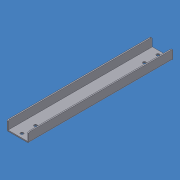
# Autodesk Inventor part: schuivend U-profiel L340
Saved by Autodesk Inventor 2015 SP1 (Build 190203100, 203)
## iProperties
Created: 2007-07-03
Part Number: schuivend U-profiel L340
Material: Steel, Mild
Document SubType Name: Sheet Metal
Designer: kurt
Manufacturer: Standard
Standards Organization: Custom
Density: 1 g/cm^3
Sheet Metal Rule: Default
Appearance: Steel
Author: kurt
Autodesk Inventor part; units mm, degrees
ref_plane "YZ Plane" through (0, 0, 0) normal (1, 0, 0) x (0, 1, 0)
ref_plane "XZ Plane" through (0, 0, 0) normal (0, 1, 0) x (-1, 0, 0)
ref_plane "XY Plane" through (0, 0, 0) normal (0, 0, 1) x (1, 0, 0)
sketch "Sketch1" plane through (0, 0, 0) normal (0, 0, 1) x (1, 0, 0)
  line L0 (-36, 0) -> (36, 0)
  line L1 (36, 0) -> (36, 530)
  line L2 (36, 530) -> (-36, 530)
  line L3 (-36, 530) -> (-36, 0)
  point P0 (0, 0)
  point P1 (0, 0)
  dimension "d2" = 72
  dimension "d3" = 530
  measures "d2" distance of L0.start L0.end
  measures "d3" distance of L0.end L1.end
extrude "Plate1" add sketch "Sketch1" along normal blind 4
sketch "Sketch2" plane through (-36, 0, 4) normal (1, 0, 0) x (0, 1, 0)
  line L0 (0, 0) -> (530, 0)
  line L1 (530, 0) -> (530, 31)
  line L2 (530, 31) -> (0, 31)
  line L3 (0, 31) -> (0, 0)
  constraints: 6 end point, 1 horizontal, 1 perpendicular, 1 vertical
sheet face with bend "Flange1" sketch "Sketch2" thickness 4 toward (-1, 0, 0) bend radius 0.001 relief straight relief width 4 relief depth 0.001
bend "Bend1"
sketch "Sketch3" plane through (36, 530, 4) normal (-1, 0, 0) x (0, -1, 0)
  line L0 (0, 0) -> (530, 0)
  line L1 (530, 0) -> (530, 31)
  line L2 (530, 31) -> (0, 31)
  line L3 (0, 31) -> (0, 0)
  constraints: 6 end point, 1 horizontal, 1 perpendicular, 1 vertical
sheet face with bend "Flange2" sketch "Sketch3" thickness 4 toward (1, 0, 0) bend radius 0.001 relief straight relief width 4 relief depth 0.001
bend "Bend2"
sketch "Sketch4" plane through (-35.999, 0, 0) normal (0, 0, -1) x (-1, 0, 0)
  line L0 (-71.998, 530) -> (0, 530) projected
  circle A0 centre (-35.999, 515) radius 5.5
  circle A1 centre (-35.999, 465) radius 5.5
  line L1 (-35.999, -53) -> (-35.999, 689) projected
  dimension "d19" = 11
  dimension "d20" = 11
  dimension "d21" = 15
  dimension "d22" = 50
  constraints: 2 centre point, 2 point on line
  measures "d19" diameter of A0
  measures "d20" diameter of A1
  measures "d21" distance from line of L0 A0.centre
  measures "d22" distance of A1.centre A0.centre
extrude "Cut1" cut sketch "Sketch4" against normal up to next
ref_plane "Work Plane1" through (-35.999, 265, 0) normal (0, 1, 0) x (-1, 0, 0)
mirror "Mirror1" about plane through (-35.999, 265, 0) normal (0, 1, 0) of "Cut1"
fillet "Corner Round1" radius 5 4 edges at (38, 0, 35) (-38, 0, 35) (-38, 530, 35) (38, 530, 35)
ref_plane "Work Plane2" through (0, 530, 4) normal (1, 0, 0) x (0, 0, -1)
equation "\"d5\" = BendReliefWidth"
equation "\"d7\" = MinimumRemnant"
equation "\"d11\" = BendRadius"
equation "\"d6\" = BendReliefDepth"
equation "\"d8\" = BendRadius"
equation "\"d12\" = BendReliefWidth"
equation "\"d14\" = MinimumRemnant"
equation "\"d18\" = BendRadius"
equation "\"d13\" = BendReliefDepth"
equation "\"d15\" = BendRadius"
equation "\"BendReliefWidth\" = Thickness"
equation "\"CornerReliefSize\" = 4 * Thickness"
equation "\"MinimumRemnant\" = 2 * Thickness"
equation "\"TransitionRadius\" = BendRadius"
equation "\"d4\" = BendRadius"
equation "\"JacobiRadiusSize\" = Thickness"
equation "\"GapSize\" = Thickness"
equation "\"BendRadius\" = 0.001"
equation "\"BendReliefDepth\" = 0.001"
equation "\"Thickness\" = 4"
body "Solid1"
